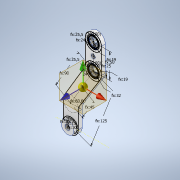
# Autodesk Inventor part: ParallelSystem_ProximalPart_Driven_Counterpart_v2.1_Rillenkugellager
Saved by Autodesk Inventor 2022 (Build 260153000, 153)
## iProperties
Created: 2022-07-18
Part Number: ParallelSystem_ProximalPart_Driven_Counterpart_v2.1_Rillenkugellager
Material: Aluminium 6061
Document SubType Name: Modeling
Designer: alexw
Density: 2.7 g/cm^3
Appearance: Aluminium - flach
Mass: 121.645 g
Surface Area: 167.633 cm^2
Volume: 45.0538 cm^3
d0: 10,000 mm
d1: 25,000 mm
d4: 30,000 mm
d7: 5,000 mm
d8: 0,00 grd
d9: 6,000 mm
d10: 0,00 grd
d11: 25,000 mm
d23: 8,000 mm
d36: 0,00 grd
d37: 30,000 mm
d38: 60,00 grd
d40: 90,000 mm
d41: 50,000 mm
d42: 45,000 mm
d43: 19,000 mm
d44: 12,000 mm
d45: 25,000 mm
Passfeder_width: 3,000 mm
Nabennuttiefe: 1,400 mm
d51: 3,000 mm
d52: 1,400 mm
ParallelLink_BearingStep_Height: 6,000 mm
ParallelLink_Lever_Thickness: 8,000 mm
ParallelHebel_Gabelgelenk_OuterDia: 32,000 mm
Nadellager_OuterDia: 19,000 mm
ParallelHebel_Passflansch_HoleDia: 25,500 mm
Author: alexw
Autodesk Inventor part; units mm, degrees
ref_plane "YZ Plane" through (0, 0, 0) normal (1, 0, 0) x (0, 1, 0)
ref_plane "XZ Plane" through (0, 0, 0) normal (0, 1, 0) x (-1, 0, 0)
ref_plane "XY Plane" through (0, 0, 0) normal (0, 0, 1) x (1, 0, 0)
sketch "Skizze1" plane through (0, 0, 0) normal (0, 0, 1) x (1, 0, 0)
  arc A0 (-1.5, 4.7697) -> (1.5, 4.7697) centre (0, 0) ccw
  circle A1 centre (0, 0) radius 12.5
  line L0 (-30.9429, 0) -> (77.0229, 0) construction
  circle A2 centre (0, 0) radius 15
  circle A3 centre (45, 116.619) radius 16
  line L1 (61, 116.619) -> (61, 166.619)
  line L2 (29, 116.619) -> (29, 166.619)
  line L3 (45, 116.619) -> (45, 182.619) construction
  line L4 (45, 116.619) -> (45, 132.619) construction
  line L5 (29, 116.619) -> (61, 116.619) construction
  line L6 (-15, 0) -> (-15, 38.6768)
  line L7 (15, 0) -> (15, 38.6768)
  line L8 (-15, 38.6768) -> (15, 38.6768) construction
  circle A4 centre (0, 38.6768) radius 15 construction
  line L9 (-12.8844, 46.3574) -> (29, 116.619)
  arc A5 (-12.8844, 46.3574) -> (-15, 38.6768) centre (0, 38.6768) ccw
  line L10 (15, 38.6768) -> (58.5544, 108.1174)
  arc A6 (58.5544, 108.1174) -> (61, 116.619) centre (45, 116.619) ccw
  line L11 (0, 38.6768) -> (45, 116.619) construction
  circle A7 centre (45, 166.619) radius 16
  circle A8 centre (45, 166.619) radius 9.5
  circle A9 centre (45, 116.619) radius 9.5
  line L12 (-1.5, 6.4) -> (1.5, 6.4)
  line L13 (1.5, 6.4) -> (1.5, 4.7697)
  line L14 (-1.5, 4.7697) -> (-1.5, 6.4)
  line L15 (0, 0) -> (0, 5) construction
  line L16 (0, 5) -> (1.5, 5) construction
  circle A10 centre (45, 116.619) radius 12.75 construction
  circle A11 centre (45, 166.619) radius 12.75 construction
  circle A12 centre (45, 116.619) radius 10.5
  circle A13 centre (45, 166.619) radius 10.5
  circle A14 centre (45, 116.619) radius 12
  circle A15 centre (45, 166.619) radius 12
  point P0 (22.5, 77.6479)
  point P1 (45, 141.619)
  point P2 (-13, 0)
  point P3 (13, 0)
  point P4 (0, 6.4)
  point P5 (45, 129.369)
  point P6 (33.9582, 110.244)
  point P7 (56.0418, 110.244)
  point P8 (45, 179.369)
  point P9 (33.9582, 160.244)
  point P10 (56.0418, 160.244)
  dimension "d69" = 25.5
  dimension "ParallelHebel_Passflansch_HoleDia" = 25.5
  dimension "d0" = 10
  dimension "d1" = 25
  dimension "d4" = 30
  dimension "d36" = 0
  dimension "ParallelHebel_Gabelgelenk_OuterDia" = 32
  dimension "d38" = 60
  dimension "d40" = 90
  dimension "d41" = 50
  dimension "d42" = 45
  dimension "d43" = 19
  dimension "Nadellager_OuterDia" = 19
  dimension "d45" = 25
  dimension "d51" = 3
  dimension "d52" = 1.4
  dimension "d67" = 360
  dimension "d72" = 360
  dimension "d83" = 21
  dimension "d84" = 24
  dimension "d85" = 21
  dimension "d86" = 24
  dimension "d91" = 125
  constraints: 32 end point, 17 point on circle, 14 centre point, 13 tangent, 12 coincident, 10 point on line, 5 perpendicular, 4 midpoint, 2 equal radius, 2 horizontal, 2 parallel, 2 vertical, 2 vertical alignment, 12 other
  measures "d0" diameter of A0
  measures "d1" diameter of A1
  measures "d4" diameter of A2
  measures "d36" distance between parallel lines of L3 L4
  measures "ParallelHebel_Gabelgelenk_OuterDia" diameter of A3
  measures "d38" angle of L8 L11
  measures "d40" distance of point (45, 116.619) A4.centre
  measures "d41" distance of A7.centre point (45, 116.619)
  measures "d42" distance of point (22.5, 77.648) A4.centre
  measures "d43" diameter of A8
  measures "Nadellager_OuterDia" diameter of A9
  measures "d45" distance of point (45, 141.619) point (45, 116.619)
  measures "d51" distance of L12.start L12.end
  measures "d52" distance between parallel lines of L12 L16
  measures "d83" diameter of A12
  measures "d84" diameter of A14
  measures "d85" diameter of A13
  measures "d86" diameter of A15
  measures "d91" distance of A3.centre point (0, 0)
extrude "Extrusion1" add sketch "Skizze1" along normal blind 6 contours A1
extrude "Extrusion2" add sketch "Skizze1" against normal blind 8 contours A1 | A2 | A2 L6 A5 L9 A3 L10 L7 | A3 | L2 A7 L1 A3 | A7 | A12 | A13 | A14 | A15
fillet "Rundung1" radius 25 2 edges at (29, 116.619, -4) (15, 38.6768, -4)
hole "Bohrung2" at (45, 141.619, 0) at (22.5, 77.6479, 0) direction (0, 0, -1) diameter 8 end through all
ref_plane "Arbeitsebene1" through (45, 116.619, 0) normal (1, 0, 0) x (0, 0, -1)
extrude "Extrusion5" cut sketch "Skizze1" against normal blind 1 contours A12 | A13 | A14 | A15
extrude "Extrusion6" cut sketch "Skizze1" against normal blind 1 from surface at -1 contours A12 | A13
equation "\"d1_1\" = 25"
equation "\"d8_1\" = 0"
equation "\"d10_1\" = 0"
equation "\"d11_1\" = 25"
equation "\"d23_1\" = 8"
equation "\"d36_1\" = 0"
equation "\"d38_1\" = 60deg"
equation "\"d39_1\" = 35"
equation "\"ParallelLink_Lever_Thickness_1\" = 14"
equation "\"ParallelHebel_Gabelgelenk_OuterDia_1\" = 32"
equation "\"Nadellager_OuterDia_1\" = 19"
equation "\"ParallelHebel_Passflansch_HoleDia_1\" = 25.5"
equation "\"d39_1_2\" = 35"
